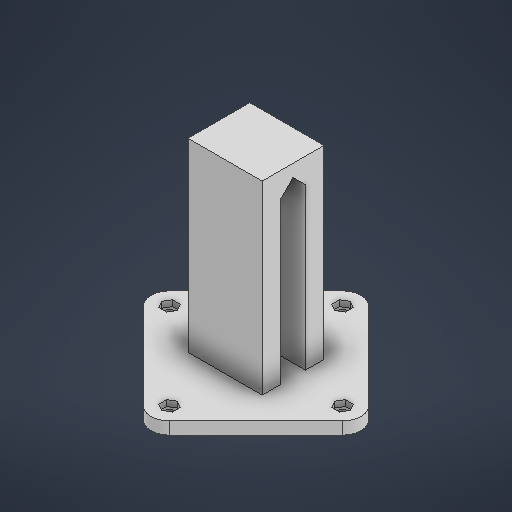
# Autodesk Inventor part: turning prevention
Saved by Autodesk Inventor 2025.2 (Build 292293000, 293)
## iProperties
Created: 2025-05-21
Part Number: turning prevention
Material: Generic
Document SubType Name: Modeling
Designer: klawy
Density: 1 g/cm^3
Appearance: Default
Author: klawy
Autodesk Inventor part; units mm, degrees
ref_plane "YZ Plane" through (0, 0, 0) normal (1, 0, 0) x (0, 1, 0)
ref_plane "XZ Plane" through (0, 0, 0) normal (0, 1, 0) x (-1, 0, 0)
ref_plane "XY Plane" through (0, 0, 0) normal (0, 0, 1) x (1, 0, 0)
sketch "Sketch1" plane through (0, 0, 0) normal (0, 1, 0) x (-1, 0, 0)
  circle A0 centre (0, 0) radius 17.5 construction
  line L0 (0, 35) -> (0, -35) construction
  line L1 (35, 0) -> (-35, 0) construction
  dimension "d0" = 35
  dimension "d1" = 70
  dimension "d2" = 70
  constraints: 5 coincident, 4 end point, 2 midpoint, 1 centre point, 1 horizontal, 1 vertical
  measures "d0" diameter of A0
  measures "d1" distance of L1.start L1.end
  measures "d2" distance of L0.start L0.end
sketch "Sketch2" plane through (0, 0, 0) normal (0, 1, 0) x (-1, 0, 0)
  circle A0 centre (0, 0) radius 17.5 construction
  line L0 (0, 35) -> (0, -35) construction
  line L1 (35, 0) -> (-35, 0) construction
  circle A1 centre (35, 0) radius 7.5
  circle A2 centre (0, 35) radius 7.5
  circle A3 centre (-35, 0) radius 7.5
  circle A4 centre (0, -35) radius 7.5
  line L2 (5.3033, 40.3033) -> (40.3033, 5.3033)
  line L3 (-40.3033, 5.3033) -> (-5.3033, 40.3033)
  line L4 (-5.3033, -40.3033) -> (-40.3033, -5.3033)
  line L5 (40.3033, -5.3033) -> (5.3033, -40.3033)
  circle A5 centre (0, 0) radius 2.5
  point P0 (5.3033, -40.3033)
  point P1 (-40.3033, -5.3033)
  dimension "d3" = 15
  dimension "d6" = 360
  dimension "d10" = 360
  dimension "d14" = 5
  constraints: 8 end point, 3 centre point, 2 coincident, 30 other
  measures "d14" diameter of A5
extrude "Extrusion1" add sketch "Sketch2" against normal blind 5
hole "Hole1" at (0, 0, -35) at (0, 0, 35) at (-35, 0, 0) at (35, 0, 0) direction (0, -1, 0) diameter 3.4 end through all clearance for "Socket Head Cap Screw ISO 4762" size "M3" standard "ISO"
sketch "Sketch3" plane through (0, 0, 0) normal (0, 1, 0) x (1, 0, 0)
  line L0 (15, -12.5) -> (-15, -12.5)
  line L1 (-15, -12.5) -> (-15, 12.5)
  line L2 (-15, 12.5) -> (15, 12.5)
  line L3 (15, 12.5) -> (15, -12.5)
  circle A0 centre (0, 0) radius 2.5 projected
  line L4 (15, -12.5) -> (-15, 12.5) construction
  line L5 (-15, -12.5) -> (15, 12.5) construction
  line L6 (15, -5) -> (-15, -5)
  line L7 (-15, -5) -> (-15, 5)
  line L8 (-15, 5) -> (15, 5)
  line L9 (15, 5) -> (15, -5)
  line L10 (15, -5) -> (-15, 5) construction
  line L11 (-15, -5) -> (15, 5) construction
  point P0 (15, -5)
  dimension "d22" = 30
  dimension "d23" = 25
  dimension "d24" = 10
  constraints: 24 end point, 4 midpoint, 4 parallel, 2 horizontal, 2 perpendicular, 1 point on line
  measures "d22" distance of L1.end L2.end
  measures "d23" distance of L0.end L1.end
  measures "d24" distance between parallel lines of L6 L8
extrude "Extrusion2" add sketch "Sketch3" along normal blind 70 contours L0 L1 L6 L3 | L8 L1 L2 L3
sketch "Sketch4" plane through (0, 70, 0) normal (0, 1, 0) x (1, 0, 0)
  line L0 (-15, 12.5) -> (15, 12.5)
  line L1 (15, 12.5) -> (15, -12.5)
  line L2 (15, -12.5) -> (-15, -12.5)
  line L3 (-15, -12.5) -> (-15, 12.5)
  point P0 (0, 0)
  constraints: 8 end point, 2 parallel, 1 horizontal, 1 perpendicular
extrude "Extrusion3" add sketch "Sketch4" along normal blind 5
sketch "Sketch5" plane through (0, 0, 0) normal (0, 1, 0) x (1, 0, 0)
  line L0 (15, -12.5) -> (-15, -12.5) projected
  line L1 (-15, -12.5) -> (-15, -5) projected
  line L2 (-15, -5) -> (15, -5) projected
  line L3 (15, -5) -> (15, -12.5) projected
  line L4 (-15, 12.5) -> (15, 12.5) projected
  line L5 (15, 12.5) -> (15, 5) projected
  line L6 (15, 5) -> (-15, 5) projected
  line L7 (-15, 5) -> (-15, 12.5) projected
  circle A0 centre (35, 0) radius 1.7 projected
  circle A1 centre (-35, 0) radius 1.7 projected
  circle A2 centre (0, -35) radius 1.7 projected
  circle A3 centre (0, 35) radius 1.7 projected
  arc A4 (-40.3033, 5.3033) -> (-40.3033, -5.3033) centre (-35, 0) ccw projected
  line L8 (-40.3033, -5.3033) -> (-5.3033, -40.3033) projected
  arc A5 (-5.3033, -40.3033) -> (5.3033, -40.3033) centre (0, -35) ccw projected
  line L9 (5.3033, -40.3033) -> (40.3033, -5.3033) projected
  arc A6 (40.3033, -5.3033) -> (40.3033, 5.3033) centre (35, 0) ccw projected
  line L10 (40.3033, 5.3033) -> (5.3033, 40.3033) projected
  arc A7 (5.3033, 40.3033) -> (-5.3033, 40.3033) centre (0, 35) ccw projected
  line L11 (-5.3033, 40.3033) -> (-40.3033, 5.3033) projected
  circle A8 centre (0, 0) radius 2.5 projected
  circle A9 centre (-35, 0) radius 2.75 construction
  line L12 (-33.4123, 2.75) -> (-31.8246, 0)
  line L13 (-31.8246, 0) -> (-33.4123, -2.75)
  line L14 (-33.4123, -2.75) -> (-36.5877, -2.75)
  line L15 (-36.5877, -2.75) -> (-38.1754, 0)
  line L16 (-38.1754, 0) -> (-36.5877, 2.75)
  line L17 (-36.5877, 2.75) -> (-33.4123, 2.75)
  line L18 (-2.75, -33.4123) -> (0, -31.8246)
  line L19 (0, -31.8246) -> (2.75, -33.4123)
  circle A10 centre (0, -35) radius 2.75 construction
  line L20 (0, -38.1754) -> (-2.75, -36.5877)
  line L21 (2.75, -36.5877) -> (0, -38.1754)
  line L22 (2.75, -33.4123) -> (2.75, -36.5877)
  line L23 (-2.75, -36.5877) -> (-2.75, -33.4123)
  line L24 (33.4123, -2.75) -> (31.8246, 0)
  line L25 (31.8246, 0) -> (33.4123, 2.75)
  circle A11 centre (35, 0) radius 2.75 construction
  line L26 (38.1754, 0) -> (36.5877, -2.75)
  line L27 (36.5877, 2.75) -> (38.1754, 0)
  line L28 (33.4123, 2.75) -> (36.5877, 2.75)
  line L29 (36.5877, -2.75) -> (33.4123, -2.75)
  line L30 (2.75, 33.4123) -> (0, 31.8246)
  line L31 (0, 31.8246) -> (-2.75, 33.4123)
  circle A12 centre (0, 35) radius 2.75 construction
  line L32 (0, 38.1754) -> (2.75, 36.5877)
  line L33 (-2.75, 36.5877) -> (0, 38.1754)
  line L34 (-2.75, 33.4123) -> (-2.75, 36.5877)
  line L35 (2.75, 36.5877) -> (2.75, 33.4123)
  point P0 (-35, 2.75)
  point P1 (-2.75, -35)
  point P2 (35, -2.75)
  point P3 (2.75, 35)
  dimension "d29" = 5.5
  dimension "d32" = 360
  constraints: 48 end point, 8 coincident, 2 horizontal alignment, 2 vertical alignment, 1 horizontal, 1 midpoint, 94 other
extrude "Extrusion4" cut sketch "Sketch5" against normal blind 2.4 contours A0 | A1 | A2 | L12 L13 L14 L15 L16 L17 | L18 L19 L22 L21 L20 L23 | L24 L25 L28 L27 L26 L29 | L30 L31 L34 L33 L32 L35
chamfer "Chamfer1" distance 5 angle 45 2 edges at (0, 70, -5) (0, 70, 5)
body "Solid1"
